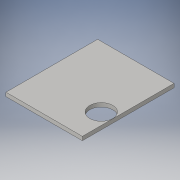
# Autodesk Inventor part: Side_chasis
Saved by Autodesk Inventor 2016 (Build 200138000, 138)
## iProperties
Created: 2016-02-28
Part Number: Side_chasis
Material: Generic
Document SubType Name: Modeling
Designer: torti_000
Density: 1 g/cm^3
Appearance: Default
Author: torti_000
Autodesk Inventor part; units mm, degrees
ref_plane "YZ Plane" through (0, 0, 0) normal (1, 0, 0) x (0, 1, 0)
ref_plane "XZ Plane" through (0, 0, 0) normal (0, 1, 0) x (-1, 0, 0)
ref_plane "XY Plane" through (0, 0, 0) normal (0, 0, 1) x (1, 0, 0)
sketch "Sketch1" plane through (0, 0, 0) normal (0, 1, 0) x (-1, 0, 0)
  line L0 (0, 0) -> (0, -152.4)
  line L1 (0, -152.4) -> (127, -152.4)
  line L2 (127, -152.4) -> (127, 0)
  line L3 (127, 0) -> (0, 0)
  dimension "d0" = 152.4
  dimension "d1" = 127
  constraints: 8 end point, 3 perpendicular, 1 vertical
  measures "d0" distance of L0.start L0.end
  measures "d1" distance of L0.end L1.end
extrude "Extrusion1" add sketch "Sketch1" along normal blind 6.35
sketch "Sketch2" plane through (0, 6.35, 0) normal (0, 1, 0) x (1, 0, 0)
  circle A0 centre (-19.3538, 50.8) radius 19.05
  point P0 (0, 0)
  dimension "d5" = 38.1
  constraints: 1 centre point
  measures "d5" diameter of A0
extrude "Extrusion2" cut sketch "Sketch2" against normal blind 6.35
body "Solid1"
